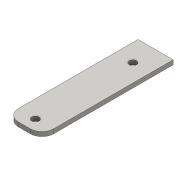
# Autodesk Inventor part: Fixação luz de freio
Saved by Autodesk Inventor 2016 (Build 200138000, 138)
## iProperties
Created: 2019-02-04
Part Number: Fixação luz de freio
Material: Genérico
Document SubType Name: Modeling
Designer: Usuario
Density: 1 g/cm^3
Appearance: Padrão
Author: Usuario
Autodesk Inventor part; units mm, degrees
ref_plane "YZ Plane" through (0, 0, 0) normal (1, 0, 0) x (0, 1, 0)
ref_plane "XZ Plane" through (0, 0, 0) normal (0, 1, 0) x (-1, 0, 0)
ref_plane "XY Plane" through (0, 0, 0) normal (0, 0, 1) x (1, 0, 0)
sketch "Esboço1" plane through (0, 0, 0) normal (0, 0, 1) x (1, 0, 0)
  line L0 (0, 0) -> (81.5, 0)
  line L1 (0, 0) -> (-2.5, 0)
  circle A0 centre (-2.5, 0) radius 2.5
  line L2 (-2.5, 0) -> (-2.5, 2.5)
  line L3 (-2.5, 2.5) -> (-2.5, 64)
  line L4 (-2.5, 64) -> (-2.5, 66.5)
  circle A1 centre (-2.5, 66.5) radius 2.5
  line L5 (-2.5, -2.5) -> (-2.5, -7.5)
  line L6 (-14.5, 7.5) -> (-14.5, 0.5)
  line L7 (-6.5, -7.5) -> (1.5, -7.5)
  line L8 (9.5, 0.5) -> (9.5, 7.5)
  line L9 (9.5, 7.5) -> (-14.5, -7.5) construction
  line L10 (-14.5, 7.5) -> (9.5, -7.5) construction
  arc A2 (-14.5, 0.5) -> (-6.5, -7.5) centre (-6.5, 0.5) ccw
  arc A3 (1.5, -7.5) -> (9.5, 0.5) centre (1.5, 0.5) ccw
  line L11 (40.75, 0) -> (40.75, 71.7729)
  line L12 (-14.5, 7.5) -> (-14.5, 82)
  line L13 (-2.5, 69) -> (-2.5, 74)
  line L14 (9.5, 7.5) -> (9.5, 82)
  line L15 (-14.5, 82) -> (9.5, 82)
  dimension "d7" = 5
  dimension "d0" = 81.5
  dimension "d3" = 5
  dimension "d5" = 61.5
  dimension "d6" = 2.5
  dimension "d11" = 5
  dimension "d13" = 24
  dimension "d14" = 8
  dimension "d15" = 8
  dimension "d16" = 5
  dimension "d17" = 8
  constraints: 32 end point, 6 point on circle, 6 point on line, 6 vertical, 4 tangent, 3 centre point, 3 horizontal, 3 midpoint, 2 coincident, 1 parallel, 1 vertical alignment, 2 other
  measures "d0" distance of L0.start L0.end
  measures "d3" diameter of A0
  measures "d5" distance of L2.end L3.end
  measures "d6" distance of L3.end L4.end
  measures "d11" distance of L5.start L5.end
  measures "d13" distance of L10.end L9.end
  measures "d14" radius of A2
  measures "d15" radius of A3
  measures "d16" distance of L13.start L13.end
  measures "d17" vertical distance of L12.end L13.end
extrude "Extrusão1" add sketch "Esboço1" along normal blind 3 contours A0 L5 L7 A2 L6 L12 L15 L14 L8 A3 L0 | L0 A3 L7 L5 A0
